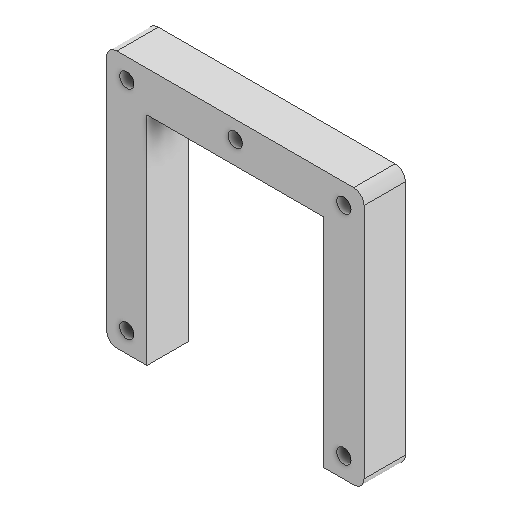
# Autodesk Inventor part: 00_Linear_Stage_NEMA11_Mount_Lid
Saved by Autodesk Inventor 2022 (Build 260153000, 153)
## iProperties
Created: 2022-02-11
Part Number: 00_Linear_Stage_NEMA11_Mount_Lid
Material: Generic
Document SubType Name: Modeling
Designer: wanghaoran
Density: 1 g/cm^3
Appearance: Default
Author: wanghaoran
Autodesk Inventor part; units mm, degrees
ref_plane "YZ Plane" through (0, 0, 0) normal (1, 0, 0) x (0, 1, 0)
ref_plane "XZ Plane" through (0, 0, 0) normal (0, 1, 0) x (-1, 0, 0)
ref_plane "XY Plane" through (0, 0, 0) normal (0, 0, 1) x (1, 0, 0)
sketch "Sketch1" plane through (0, 0, 0) normal (0, 0, 1) x (1, 0, 0)
  circle A0 centre (-21, 1.215) radius 1.4 projected
  circle A1 centre (21, 1.215) radius 1.4 projected
  arc A2 (24.9, 3.115) -> (22.9, 5.115) centre (22.9, 3.115) ccw projected
  line L0 (22.9, 5.115) -> (-22.9, 5.115) projected
  arc A3 (-22.9, 5.115) -> (-24.9, 3.115) centre (-22.9, 3.115) ccw projected
  line L1 (-24.9, 3.115) -> (-24.9, -5.115) projected
  line L2 (-24.9, -5.115) -> (24.9, -5.115) projected
  line L3 (24.9, -5.115) -> (24.9, 3.115) projected
  arc A4 (22.9, -44.685) -> (24.9, -42.685) centre (22.9, -42.685) ccw projected
  line L4 (24.9, -42.685) -> (24.9, -36.885) projected
  line L5 (24.9, -36.885) -> (17.1, -36.885) projected
  line L6 (17.1, -36.885) -> (17.1, -44.685) projected
  line L7 (17.1, -44.685) -> (22.9, -44.685) projected
  circle A5 centre (21, -40.785) radius 1.4 projected
  arc A6 (-24.9, -42.685) -> (-22.9, -44.685) centre (-22.9, -42.685) ccw projected
  line L8 (-22.9, -44.685) -> (-17.1, -44.685) projected
  line L9 (-17.1, -44.685) -> (-17.1, -36.885) projected
  line L10 (-17.1, -36.885) -> (-24.9, -36.885) projected
  line L11 (-24.9, -36.885) -> (-24.9, -42.685) projected
  circle A7 centre (-21, -40.785) radius 1.4 projected
  line L12 (24.9, 5.115) -> (-24.9, 5.115)
  line L13 (-24.9, 5.115) -> (-24.9, -44.685)
  line L14 (-24.9, -44.685) -> (24.9, -44.685)
  line L15 (24.9, -44.685) -> (24.9, 5.115)
  line L16 (17.1, -2.685) -> (-17.1, -2.685)
  line L17 (-17.1, -2.685) -> (-17.1, -36.885)
  line L18 (-17.1, -36.885) -> (17.1, -36.885)
  line L19 (17.1, -36.885) -> (17.1, -2.685)
  line L20 (17.1, -36.885) -> (17.1, -44.685)
  line L21 (-17.1, -36.885) -> (-17.1, -44.685)
  circle A8 centre (0, 1.415) radius 1.4 projected
  point P0 (0, 0)
  dimension "d0" = 7.8
  constraints: 20 end point, 6 equal length, 2 perpendicular, 1 horizontal, 1 point on line, 3 other
  measures "d0" distance between parallel lines of L15 L19
extrude "Extrusion1" add sketch "Sketch1" along normal blind 8 contours L3 L2 L19 L16 L17 L1 A3 L0 A2 | L15 L5 L19 L2 | L4 A4 L7 L6 L5 | L17 L10 L13 L2 | L9 L8 A6 L11 L10 | A8
sketch "Sketch2" plane through (0, 0, 8) normal (0, 0, 1) x (1, 0, 0)
  circle A0 centre (0, 1.715) radius 1.4
  line L0 (22.9, 5.115) -> (-22.9, 5.115) projected
  point P0 (0, 0)
  dimension "d3" = 2.8
  dimension "d4" = 3.4
  constraints: 1 centre point
  measures "d3" diameter of A0
  measures "d4" distance from line of L0 A0.centre
extrude "Extrusion2" cut sketch "Sketch2" against normal blind 8
body "Solid1"
